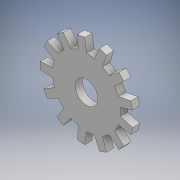
# Autodesk Inventor part: efektor zebatka1
Saved by Autodesk Inventor 2017.3 (Build 213256000, 256)
## iProperties
Created: 2019-03-17
Part Number: efektor zebatka1
Material: Ogólny
Document SubType Name: Modeling
Designer: legox
Density: 1 g/cm^3
Appearance: Domyślna
Author: legox
Autodesk Inventor part; units mm, degrees
ref_plane "YZ Plane" through (0, 0, 0) normal (1, 0, 0) x (0, 1, 0)
ref_plane "XZ Plane" through (0, 0, 0) normal (0, 1, 0) x (-1, 0, 0)
ref_plane "XY Plane" through (0, 0, 0) normal (0, 0, 1) x (1, 0, 0)
sketch "Szkic2" plane through (0, 0, 0) normal (0, 1, 0) x (-1, 0, 0)
  circle A0 centre (0, 0) radius 2.5
  circle A1 centre (0, 0) radius 10.25
  line L0 (10.2187, -0.8002) -> (10.2187, 0.8002)
  line L1 (10.2187, -0.8002) -> (7.4401, -0.9459)
  line L2 (10.2187, -0.8002) -> (13.0011, -0.8002) construction
  line L3 (10.2187, 0.8002) -> (7.4401, 0.9459)
  line L4 (10.2187, 0.8002) -> (13.0011, 0.8002) construction
  line L5 (9.4201, 4.0403) -> (7.0275, 2.6201)
  line L6 (8.6763, 5.4575) -> (6.1483, 4.2951)
  line L7 (9.4201, 4.0403) -> (8.6763, 5.4575)
  line L8 (6.4635, 7.9552) -> (5.0049, 5.5858)
  line L9 (5.1463, 8.8644) -> (3.448, 6.6604)
  line L10 (6.4635, 7.9552) -> (5.1463, 8.8644)
  line L11 (2.0261, 10.0477) -> (1.8358, 7.2719)
  line L12 (0.4373, 10.2407) -> (-0.0422, 7.4999)
  line L13 (2.0261, 10.0477) -> (0.4373, 10.2407)
  line L14 (-2.8754, 9.8384) -> (-1.7539, 7.292)
  line L15 (-4.3718, 9.2709) -> (-3.5227, 6.6212)
  line L16 (-2.8754, 9.8384) -> (-4.3718, 9.2709)
  line L17 (-7.1182, 7.3753) -> (-4.9418, 5.6417)
  line L18 (-8.1795, 6.1773) -> (-6.1962, 4.2257)
  line L19 (-7.1182, 7.3753) -> (-8.1795, 6.1773)
  line L20 (-9.7303, 3.2225) -> (-6.9976, 2.6989)
  line L21 (-10.1133, 1.6685) -> (-7.4503, 0.8622)
  line L22 (-9.7303, 3.2225) -> (-10.1133, 1.6685)
  line L23 (-10.1133, -1.6685) -> (-7.4503, -0.8622)
  line L24 (-9.7303, -3.2225) -> (-6.9976, -2.6989)
  line L25 (-10.1133, -1.6685) -> (-9.7303, -3.2225)
  line L26 (-8.1795, -6.1773) -> (-6.1962, -4.2257)
  line L27 (-7.1182, -7.3753) -> (-4.9418, -5.6417)
  line L28 (-8.1795, -6.1773) -> (-7.1182, -7.3753)
  line L29 (-4.3718, -9.2709) -> (-3.5227, -6.6212)
  line L30 (-2.8754, -9.8384) -> (-1.7539, -7.292)
  line L31 (-4.3718, -9.2709) -> (-2.8754, -9.8384)
  line L32 (0.4373, -10.2407) -> (-0.0422, -7.4999)
  line L33 (2.0261, -10.0477) -> (1.8358, -7.2719)
  line L34 (0.4373, -10.2407) -> (2.0261, -10.0477)
  line L35 (5.1463, -8.8644) -> (3.448, -6.6604)
  line L36 (6.4635, -7.9552) -> (5.0049, -5.5858)
  line L37 (5.1463, -8.8644) -> (6.4635, -7.9552)
  line L38 (8.6763, -5.4575) -> (6.1483, -4.2951)
  line L39 (9.4201, -4.0403) -> (7.0275, -2.6201)
  line L40 (8.6763, -5.4575) -> (9.4201, -4.0403)
  arc A2 (7.0275, -2.6201) -> (7.4401, -0.9459) centre (0, 0) ccw
  arc A3 (5.0049, -5.5858) -> (6.1483, -4.2951) centre (0, 0) ccw
  arc A4 (7.4401, 0.9459) -> (7.0275, 2.6201) centre (0, 0) ccw
  arc A5 (6.1483, 4.2951) -> (5.0049, 5.5858) centre (0, 0) ccw
  arc A6 (3.448, 6.6604) -> (1.8358, 7.2719) centre (0, 0) ccw
  arc A7 (-0.0422, 7.4999) -> (-1.7539, 7.292) centre (0, 0) ccw
  arc A8 (-3.5227, 6.6212) -> (-4.9418, 5.6417) centre (0, 0) ccw
  arc A9 (-6.1962, 4.2257) -> (-6.9976, 2.6989) centre (0, 0) ccw
  arc A10 (-7.4503, 0.8622) -> (-7.4503, -0.8622) centre (0, 0) ccw
  arc A11 (-6.9976, -2.6989) -> (-6.1962, -4.2257) centre (0, 0) ccw
  arc A12 (-4.9418, -5.6417) -> (-3.5227, -6.6212) centre (0, 0) ccw
  arc A13 (-1.7539, -7.292) -> (-0.0422, -7.4999) centre (0, 0) ccw
  arc A14 (1.8358, -7.2719) -> (3.448, -6.6604) centre (0, 0) ccw
  dimension "d58" = 5
  dimension "d60" = 20.5
  dimension "d61" = 177
  dimension "d62" = 177
  dimension "d65" = 360
  constraints: 82 end point, 28 point on circle, 15 centre point, 3 coincident, 2 equal length, 2 horizontal, 1 vertical, 92 other
  measures "d58" diameter of A0
  measures "d60" diameter of A1
  measures "d61" angle of L1 L2
  measures "d62" angle of L4 L3
extrude "Wyciągnięcie proste6" add sketch "Szkic2" along normal blind 1.6 contours L0 L1 A2 L39 L40 L38 A3 L36 L37 L35 A14 L33 L34 L32 A13 L30 L31 L29 A12 L27 L28 L26 A11 L24 L25 L23 A10 L21 L22 L20 A9 L18 L19 L17 A8 L15 L16 L14 A7 L12 L13 L11 A6 L9 L10 L8 A5 L6 L7 L5 A4 L3
